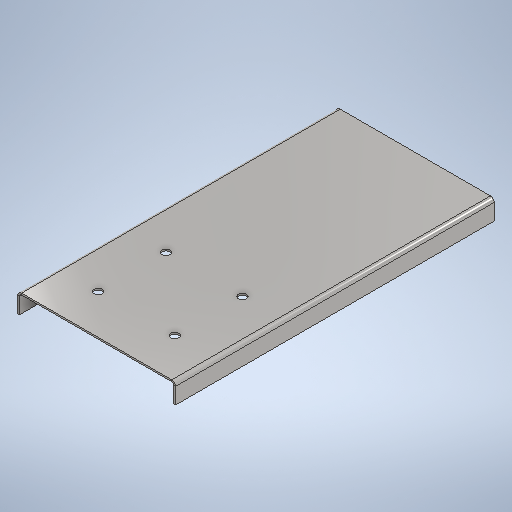
# Autodesk Inventor part: Крепление
Saved by Autodesk Inventor 2025 (Build 290162010, 162A)
## iProperties
Created: 2024-04-09
Part Number: Крепление
Material: Stainless Steel
Document SubType Name: Sheet Metal
Designer: pokla
Density: 8 g/cm^3
Sheet Metal Rule: AISI304 2mm Die16
Appearance: Semi-Polished
Flat Pattern Width: 24.0404 cm
Flat Pattern Length: 40 cm
Flat Pattern Area: 961.616 cm^2
Sheet Metal Width: 240,404 mm
Sheet Metal Length: 400,000 mm
Sheet Metal Area: 96161,593 mm^2
Stock Number: Крепление
Author: pokla
Autodesk Inventor part; units mm, degrees
ref_plane "YZ Plane" through (0, 0, 0) normal (1, 0, 0) x (0, 1, 0)
ref_plane "XZ Plane" through (0, 0, 0) normal (0, 1, 0) x (-1, 0, 0)
ref_plane "XY Plane" through (0, 0, 0) normal (0, 0, 1) x (1, 0, 0)
sketch "Sketch4" plane through (0, 0, 0) normal (0, 1, 0) x (-1, 0, 0)
  line L0 (99, -200) -> (-99, -200)
  line L1 (-99, -200) -> (-99, 200)
  line L2 (-99, 200) -> (99, 200)
  line L3 (99, 200) -> (99, -200)
  line L4 (99, -200) -> (-99, 200) construction
  point P0 (0, 0)
  point P1 (0, 0)
  dimension "d24" = 198
  dimension "d25" = 400
  measures "d24" distance of L1.end L2.end
  measures "d25" distance of L0.end L1.end
extrude "Plate4" add sketch "Sketch4" along normal mid plane 2
sketch "Sketch7" plane through (0, -1, 0) normal (0, -1, 0) x (1, 0, 0)
  circle A0 centre (48, 65) radius 5
  line L0 (99, 200) -> (99, -200) projected
  line L1 (99, -200) -> (-99, -200) projected
  line L2 (0, -200) -> (0, 200) construction
  line L3 (99, 0) -> (-99, 0) construction
  circle A1 centre (-48, 65) radius 5
  circle A2 centre (48, 150) radius 5
  circle A3 centre (-48, 150) radius 5
  line L4 (99, 200) -> (-99, 200) projected
  point P0 (0, 0)
  point P1 (0, 0)
  dimension "d41" = 10
  dimension "d46" = 85
  dimension "d57" = 96
  dimension "d70" = 135
  constraints: 4 centre point, 4 end point, 4 midpoint, 2 equal radius, 2 vertical alignment, 1 coincident, 1 horizontal, 1 horizontal alignment, 1 symmetric about line, 1 vertical, 1 other
  measures "d41" diameter of A0
  measures "d46" distance of A1.centre A3.centre
  measures "d57" distance of A0.centre A1.centre
  measures "d70" distance from line of L4 A0.centre
extrude "Extrusion2" cut sketch "Sketch7" against normal up to surface (2 mm away)
sketch "Sketch9" plane through (97, 1, -200) normal (1, 0, 0) x (0, -1, 0)
  line L0 (0, 400) -> (0, 0)
  line L1 (0, 0) -> (25, 0)
  line L2 (25, 0) -> (25, 400)
  line L3 (25, 400) -> (0, 400)
  constraints: 6 end point, 1 horizontal, 1 perpendicular, 1 vertical
edge flange "Flange5" height 25 angle 90 thickness 2 bend radius 2.75 thickness toward (1, 0, 0) relief straight relief width 2 relief depth 1 corner gap 2.75 corner form 0 edges at (99, 1, 0) (-99, 1, 0) wall of the first edge with corners at (97, 1, 200) (97, 1, -200) (97, -24, -200) (97, -24, 200)
bend "Bend5"
corner "Corner5"
sketch "Sketch12" plane through (0, 1, 0) normal (0, 1, 0) x (1, 0, 0)
  line L0 (-94.25, 200) -> (-94.25, -200) projected
  line L1 (94.25, -200) -> (-94.25, -200) projected
  line L2 (-84.125, -200) -> (-84.125, -81.7006) construction
  line L3 (-94.25, -150) -> (-26.2093, -150) construction
  circle A0 centre (-84.125, -150) radius 3
  point P0 (0, 0)
  dimension "d86" = 10.125
  dimension "d87" = 50
  dimension "d88" = 6
  constraints: 4 end point, 4 point on line, 1 centre point, 1 horizontal, 1 parallel
  measures "d86" distance between parallel lines of L0 L2
  measures "d87" distance between parallel lines of L1 L3
  measures "d88" diameter of A0
extrude "Extrusion5" [suppressed]
pattern_linear "Rectangular Pattern2" [suppressed]
equation "\"d24\" = Ширина_базовой_пластины"
equation "\"d25\" = Длина_базовой_пластины"
equation "\"d26\" = Thickness"
equation "\"d60\" = BendReliefWidth"
equation "\"d61\" = BendReliefDepth"
equation "\"d62\" = MinimumRemnant"
equation "\"d63\" = TransitionRadius"
equation "\"d66\" = BendRadius"
equation "\"d67\" = CornerReliefSize"
equation "\"d68\" = GapSize"
equation "\"d69\" = JacobiRadiusSize"
equation "\"BendReliefWidth\" = Thickness"
equation "\"BendReliefDepth\" = 0.5 * Thickness"
equation "\"CornerReliefSize\" = 4 * Thickness"
equation "\"MinimumRemnant\" = 2 * Thickness"
equation "\"TransitionRadius\" = BendRadius"
equation "\"JacobiRadiusSize\" = BendRadius"
equation "\"GapSize\" = Thickness"
equation "\"Ширина_базовой_пластины\" = 198"
equation "\"Длина_базовой_пластины\" = 400"
equation "\"Thickness\" = 2"
equation "\"BendRadius\" = 2.75"
body "Solid2"
